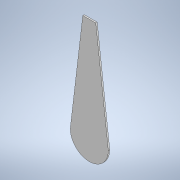
# Autodesk Inventor part: ухо
Saved by Autodesk Inventor 2021.1 (Build 251245010, 245A)
## iProperties
Created: 2023-01-27
Part Number: ухо
Material: Типовые
Document SubType Name: Modeling
Designer: zmoze
Density: 1 g/cm^3
Appearance: По умолчанию
Author: zmoze
Autodesk Inventor part; units mm, degrees
ref_plane "YZ Plane" through (0, 0, 0) normal (1, 0, 0) x (0, 1, 0)
ref_plane "XZ Plane" through (0, 0, 0) normal (0, 1, 0) x (-1, 0, 0)
ref_plane "XY Plane" through (0, 0, 0) normal (0, 0, 1) x (1, 0, 0)
sketch "Эскиз1" plane through (0, 0, 0) normal (0, 0, 1) x (1, 0, 0)
  circle A0 centre (0, 0) radius 40
  line L0 (-40, 0) -> (-13.6038, 219.402)
  line L1 (-13.6038, 219.402) -> (13.6038, 219.402)
  line L2 (13.6038, 219.402) -> (40, 0)
  line L3 (0, 0) -> (0, 40) construction
  line L4 (0, 0) -> (40, 0) construction
  point P0 (0, 219.402)
  dimension "d0" = 80
  constraints: 10 end point, 3 point on circle, 2 horizontal, 1 centre point, 1 coincident, 1 equal length, 1 midpoint, 1 point on line, 1 vertical
  measures "d0" diameter of A0
extrude "Выдавливание1" add sketch "Эскиз1" along normal blind 3 contours L0 A0 L2 | L0 L1 L2 A0
